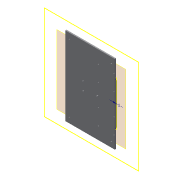
# Autodesk Inventor part: 01_Zeiss_Axiotech_adapterplate
Saved by Autodesk Inventor 2019 (Build 230136000, 136)
## iProperties
Created: 2019-05-02
Part Number: 01_Zeiss_Axiotech_adapterplate
Material: Generic
Document SubType Name: Modeling
Designer: diederichbenedict
Density: 1 g/cm^3
Appearance: Default
Author: diederichbenedict
Autodesk Inventor part; units mm, degrees
ref_plane "YZ Plane" through (0, 0, 0) normal (1, 0, 0) x (0, 1, 0)
ref_plane "XZ Plane" through (0, 0, 0) normal (0, 1, 0) x (-1, 0, 0)
ref_plane "Work Plane1" through (0, 0, 0) normal (0, 0, 1) x (1, 0, 0)
sketch "Sketch1" plane through (0, 0, 0) normal (0, 0, 1) x (1, 0, 0)
  arc A0 (80, 65) -> (65, 80) centre (65, 65) ccw projected
  line L0 (80, 65) -> (80, -65) projected
  arc A1 (65, -80) -> (80, -65) centre (65, -65) ccw projected
  line L1 (65, -80) -> (-65, -80) projected
  arc A2 (-80, -65) -> (-65, -80) centre (-65, -65) ccw projected
  line L2 (-80, -65) -> (-80, 65) projected
  arc A3 (-65, 80) -> (-80, 65) centre (-65, 65) ccw projected
  line L3 (-65, 80) -> (65, 80) projected
  line L4 (-150, -150) -> (150, -150) projected
  line L5 (150, -150) -> (150, 150) projected
  line L6 (150, 150) -> (-150, 150) projected
  line L7 (-150, 150) -> (-150, -150) projected
  line L8 (79, -65) -> (79, 65)
  arc A4 (79, 65) -> (65, 79) centre (65, 65) ccw
  line L9 (65, 79) -> (-65, 79)
  arc A5 (-65, 79) -> (-79, 65) centre (-65, 65) ccw
  line L10 (-79, 65) -> (-79, -65)
  arc A6 (-79, -65) -> (-65, -79) centre (-65, -65) ccw
  line L11 (-65, -79) -> (65, -79)
  arc A7 (65, -79) -> (79, -65) centre (65, -65) ccw
  circle A8 centre (-67, -107.5) radius 1.95 projected
  circle A9 centre (67, 107.5) radius 1.95 projected
  circle A10 centre (-67, 107.5) radius 1.95 projected
  circle A11 centre (67, -107.5) radius 1.95 projected
  point P0 (0, 0)
  dimension "d0" = 1
  constraints: 8 end point, 8 point on circle, 4 centre point, 7 other
  measures "d0" distance between parallel lines of L0 L8
ref_plane "Work Plane3" through (0, 0, 0) normal (0, 0, 1) x (1, 0, 0)
sketch "Sketch2" plane through (0, 0, 0) normal (0, 0, 1) x (1, 0, 0)
  line L0 (79, -65) -> (79, 65) projected
  arc A0 (79, 65) -> (65, 79) centre (65, 65) ccw projected
  line L1 (65, 79) -> (-65, 79) projected
  arc A1 (-65, 79) -> (-79, 65) centre (-65, 65) ccw projected
  line L2 (-79, 65) -> (-79, -65) projected
  arc A2 (-79, -65) -> (-65, -79) centre (-65, -65) ccw projected
  line L3 (-65, -79) -> (65, -79) projected
  arc A3 (65, -79) -> (79, -65) centre (65, -65) ccw projected
  line L4 (-79, -125) -> (79, -125)
  line L5 (79, -125) -> (79, 125)
  line L6 (79, 125) -> (-79, 125)
  line L7 (-79, 125) -> (-79, -125)
  line L8 (-79, -125) -> (79, 125) construction
  line L9 (79, -125) -> (-79, 125) construction
  point P0 (0, 0)
  dimension "d3" = 250
  constraints: 12 end point, 2 midpoint, 2 parallel, 1 horizontal, 1 perpendicular
  measures "d3" distance of L5.end L4.end
extrude "Extrusion2" add sketch "Sketch2" along normal blind 4
ref_plane "Work Plane2" through (-26.5401, 7.7836, 6.83) normal (0, 0, -1) x (0, 1, 0)
sketch "Sketch3" plane through (0, 0, 4) normal (0, 0, 1) x (1, 0, 0)
  arc A0 (-22.3322, 15.5836) -> (-25.0072, 11.4836) centre (-3.6319, 0.4603) ccw
  line L0 (-21.3013, 11.4836) -> (-25.0072, 11.4836)
  arc A1 (-21.3013, 11.4836) -> (-20.1013, 15.0836) centre (-21.3013, 13.4836) ccw
  line L1 (-20.1013, 15.5836) -> (-20.1013, 15.0836)
  line L2 (-22.3322, 15.5836) -> (-20.1013, 15.5836)
  circle A2 centre (-21.3013, 13.4836) radius 0.9
  circle A3 centre (6.0928, 10.7836) radius 1.575
  circle A4 centre (6.0928, 10.7836) radius 0.7
  circle A5 centre (4.2678, -11.3664) radius 1.575
  circle A6 centre (4.2678, -11.3664) radius 0.7
  circle A7 centre (-21.3013, 13.4836) radius 0.9
  circle A8 centre (-21.3013, 13.4836) radius 2
  circle A9 centre (25.4178, -3.2164) radius 0.9
  circle A10 centre (-20.4322, -13.5164) radius 0.9
  circle A11 centre (-20.4322, -13.5164) radius 2
  circle A12 centre (25.4178, -3.2164) radius 2
  point P0 (0, 0)
extrude "Extrusion3" add sketch "Sketch3" along normal up to surface (2.83 mm away) contours A8 A1 | A11 | A12
sketch "Sketch4" plane through (25.4178, -3.2164, 6.83) normal (0, 0, 1) x (1, 0, 0)
  circle A0 centre (0, 0) radius 2 projected
  circle A1 centre (0, 0) radius 0.9 projected
  point P0 (-25.4178, 3.2164)
extrude "Extrusion4" add sketch "Sketch4" along normal up to surface (1.2 mm away)
sketch "Sketch5" plane through (0, 0, 4) normal (0, 0, 1) x (1, 0, 0)
  circle A0 centre (-20.4322, -13.5164) radius 2 projected
  circle A1 centre (-20.4322, -13.5164) radius 0.9 projected
  circle A2 centre (-21.3013, 13.4836) radius 0.9 projected
  circle A3 centre (25.4178, -3.2164) radius 0.9 projected
  point P0 (0, 0)
extrude "Extrusion5" cut sketch "Sketch5" against normal through all contours A1 | A2 | A3
sketch "Sketch6" plane through (0, 0, 4) normal (0, 0, 1) x (1, 0, 0)
  circle A0 centre (76, -85) radius 1.95 projected
  circle A1 centre (26, -85) radius 1.95 projected
  circle A2 centre (26, -35) radius 1.95 projected
  circle A3 centre (76, -35) radius 1.95 projected
  circle A4 centre (76, 35) radius 1.95 projected
  circle A5 centre (26, 35) radius 1.95 projected
  circle A6 centre (76, 85) radius 1.95 projected
  circle A7 centre (26, 85) radius 1.95 projected
  point P0 (0, 0)
extrude "Extrusion6" cut sketch "Sketch6" against normal through all
sketch "Sketch7" plane through (0, 0, 0) normal (0, 0, -1) x (-1, 0, 0)
  circle A0 centre (-76, 85) radius 1.95 projected
  circle A1 centre (-76, 35) radius 1.95 projected
  circle A2 centre (-26, -35) radius 1.95 projected
  circle A3 centre (-76, -85) radius 1.95 projected
  circle A4 centre (-26, -85) radius 1.95 projected
  circle A5 centre (-76, -35) radius 1.95 projected
  circle A6 centre (-26, 35) radius 1.95 projected
  circle A7 centre (-26, 85) radius 1.95 projected
  line L0 (79, -125) -> (-79, -125) projected
  line L1 (79, 125) -> (79, -125) projected
  line L2 (-79, 125) -> (79, 125) projected
  line L3 (-79, -125) -> (-79, 125) projected
  line L4 (67, -107.5) -> (-67, -107.5)
  line L5 (-67, -107.5) -> (-67, 107.5)
  line L6 (-67, 107.5) -> (67, 107.5)
  line L7 (67, 107.5) -> (67, -107.5)
  line L8 (67, -107.5) -> (-67, 107.5) construction
  line L9 (-67, -107.5) -> (67, 107.5) construction
  point P0 (0, 0)
  dimension "d16" = 134
  dimension "d17" = 215
  constraints: 12 end point, 2 midpoint, 2 parallel, 1 coincident, 1 horizontal, 1 perpendicular
  measures "d16" distance of L5.end L6.end
  measures "d17" distance of L4.end L5.end
hole "Hole1" at (-67, 107.5, 0) at (67, 107.5, 0) at (67, -107.5, 0) at (-67, -107.5, 0) direction (0, 0, 1) diameter 3.9 depth 10 tip angle 118
body "Solid1"
